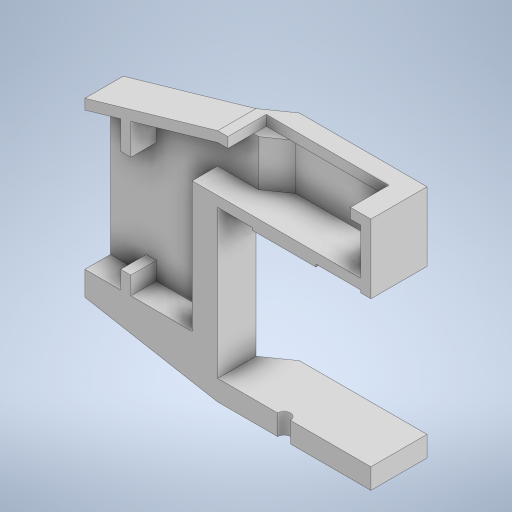
# Autodesk Inventor part: wirst 1 left
Saved by Autodesk Inventor 2023 (Build 270158000, 158)
## iProperties
Created: 2024-06-27
Part Number: wirst 1 left
Material: Generic
Document SubType Name: Modeling
Designer: Swoby
Density: 1 g/cm^3
Appearance: Default
Author: Swoby
Autodesk Inventor part; units mm, degrees
ref_plane "YZ Plane" through (0, 0, 0) normal (1, 0, 0) x (0, 1, 0)
ref_plane "XZ Plane" through (0, 0, 0) normal (0, 1, 0) x (-1, 0, 0)
ref_plane "XY Plane" through (0, 0, 0) normal (0, 0, 1) x (1, 0, 0)
sketch "Sketch1" plane through (0, 0, 0) normal (0, 0, 1) x (1, 0, 0)
  line L0 (-26, -31) -> (26, -31)
  line L1 (26, -31) -> (26, 31)
  line L2 (26, 31) -> (-26, 31)
  line L3 (-26, 31) -> (-26, -31)
  line L4 (-26, -31) -> (26, 31) construction
  line L5 (26, -31) -> (-26, 31) construction
  line L6 (-24, -23) -> (-24, -9) construction
  line L7 (-26, 31) -> (26, 46)
  line L8 (26, 46) -> (86, 46)
  line L9 (86, 46) -> (86, 19)
  line L10 (86, 19) -> (26, 19)
  point P0 (0, 0)
  dimension "d0" = 2
  dimension "d1" = 62
  dimension "d2" = 52
  dimension "d3" = 15
  dimension "d4" = 50
  dimension "d5" = 60
  constraints: 22 end point, 3 parallel, 3 perpendicular, 2 horizontal, 2 midpoint, 2 point on line
  measures "d0" distance between parallel lines of L3 L6
  measures "d1" distance of L2.end L0.start
  measures "d2" distance of L0.start L0.end
  measures "d3" distance of L1.end L7.end
  measures "d4" distance between parallel lines of L0 L10
  measures "d5" distance of L7.end L8.end
extrude "Extrusion1" add sketch "Sketch1" along normal blind 5
sketch "Sketch2" plane through (0, 0, 5) normal (0, 0, 1) x (1, 0, 0)
  line L0 (-29, 11.5) -> (-29, 6.5) construction
  line L1 (-29, 6.5) -> (-24, 6.5) construction
  line L2 (-24, 6.5) -> (-24, -20) construction
  line L3 (-24, -20) -> (-15, -20) construction
  line L4 (-15, -20) -> (-15, -27) construction
  line L5 (-15, -27) -> (-12, -27) construction
  line L6 (-12, -27) -> (-12, -20) construction
  line L7 (-12, -20) -> (16, -20) construction
  line L8 (16, -20) -> (16, 20) construction
  line L9 (16, 20) -> (11, 20) construction
  line L10 (11, 20) -> (11, 25) construction
  line L11 (11, 25) -> (8, 25) construction
  line L12 (8, 25) -> (8, 20) construction
  line L13 (8, 20) -> (-12, 20) construction
  line L14 (-12, 20) -> (-12, 27) construction
  line L15 (-12, 27) -> (-15, 27) construction
  line L16 (-15, 27) -> (-15, 20) construction
  line L17 (-15, 20) -> (-24, 20) construction
  line L18 (26, 46) -> (-26, 31) projected
  line L19 (-24, 20) -> (-24, 11.5) construction
  line L20 (-24, 11.5) -> (-29, 11.5) construction
  line L21 (-26, 31) -> (-26, -31) construction
  line L22 (-26, -31) -> (26, -31) construction
  line L23 (-12, 31.0385) -> (-12, 20)
  line L24 (-12, 20) -> (-8, 20)
  line L25 (-8, 20) -> (-8, 32.1923)
  line L26 (-26, 27) -> (26, 42)
  line L27 (-26, -27) -> (-12, -27)
  line L28 (-12, -27) -> (-12, -20)
  line L29 (-12, -20) -> (-8, -20)
  line L30 (-8, -20) -> (-8, -27)
  line L31 (-8, -27) -> (16, -27)
  line L32 (16, -27) -> (16, 20)
  line L33 (26, -31) -> (26, 19) projected
  line L34 (26, 24) -> (26, 19) construction
  line L35 (-26, 31) -> (-26, 27)
  line L36 (86, 46) -> (26, 46) projected
  line L37 (26, 46) -> (26, 42)
  line L38 (26, 42) -> (82, 42)
  line L39 (82, 42) -> (82, 19)
  line L40 (26, 19) -> (86, 19) projected
  line L41 (86, 19) -> (86, 46) projected
  line L42 (-26, -27) -> (-26, -31)
  line L43 (-26, -31) -> (26, -31)
  line L44 (16, 20) -> (16, 24)
  line L45 (16, 24) -> (26, 24)
  line L46 (26, 24) -> (82, 24)
  line L47 (26, 19) -> (26, 20)
  line L48 (26, 20) -> (82, 20)
  point P0 (0, 0)
  dimension "d8" = 3
  dimension "d9" = 3
  dimension "d10" = 3
  dimension "d11" = 7
  dimension "d12" = 54
  dimension "d13" = 7
  dimension "d14" = 5
  dimension "d15" = 5
  dimension "d16" = 2
  dimension "d17" = 9
  dimension "d18" = 8.5
  dimension "d19" = 4
  dimension "d20" = 5
  dimension "d21" = 5
  dimension "d22" = 40
  dimension "d23" = 4
  dimension "d25" = 4
  dimension "d26" = 10
  dimension "d27" = 4
  dimension "d28" = 4
  dimension "d36" = 1
  dimension "d37" = 4
  constraints: 84 end point, 16 point on line, 14 perpendicular, 12 parallel, 8 collinear, 2 horizontal, 2 vertical
  measures "d8" distance of L14.end L15.end
  measures "d9" distance of L10.end L11.end
  measures "d10" distance of L4.end L5.end
  measures "d11" distance of L15.end L16.end
  measures "d12" distance between parallel lines of L5 L15
  measures "d13" distance of L3.end L4.end
  measures "d14" distance between parallel lines of L13 L11
  measures "d15" distance of L8.end L9.end
  measures "d16" distance between parallel lines of L21 L2
  measures "d17" distance of L2.end L3.end
  measures "d18" distance of L17.end L19.end
  measures "d19" distance between parallel lines of L22 L5
  measures "d20" distance of L0.start L0.end
  measures "d21" distance of L19.end L0.start
  measures "d22" distance between parallel lines of L8 L2
  measures "d23" distance between parallel lines of L25 L23
  measures "d25" distance between parallel lines of L30 L6
  measures "d26" distance between parallel lines of L33 L32
  measures "d27" distance between parallel lines of L41 L39
  measures "d28" distance of L18.start L26.end
  measures "d36" distance of L33.end L47.end
  measures "d37" distance between parallel lines of L48 L46
extrude "Extrusion2" add sketch "Sketch2" along normal blind 10 contours L37 L26 L35 L18 | L36 L41 L40 L39 L38 L37 | L25 L24 L23 L26 | L39 L48 L47 L33 L43 L42 L27 L28 L29 L30 L31 L32 L44 L45 L46
sketch "Sketch3" plane through (0, 0, 15) normal (0, 0, 1) x (1, 0, 0)
  line L0 (-26, 27) -> (-12, 31.0385) projected
  line L1 (-12, 31.0385) -> (-12, 20) projected
  line L2 (-12, 20) -> (-8, 20) projected
  line L3 (-8, 20) -> (-8, 32.1923) projected
  line L4 (-8, 32.1923) -> (26, 42) projected
  line L5 (26, 42) -> (82, 42) projected
  line L6 (82, 42) -> (82, 24) projected
  line L7 (82, 19) -> (86, 19) projected
  line L8 (86, 19) -> (86, 46) projected
  line L9 (86, 46) -> (26, 46) projected
  line L10 (26, 46) -> (-26, 31) projected
  line L11 (-26, 31) -> (-26, 27) projected
  line L12 (30, 42) -> (78, 42)
  line L13 (78, 42) -> (78, 46)
  line L14 (78, 46) -> (30, 46)
  line L15 (30, 46) -> (30, 42)
  line L16 (82, 24) -> (16, 24) projected
  line L17 (16, 24) -> (16, -27) projected
  line L18 (16, -27) -> (-8, -27) projected
  line L19 (-8, -27) -> (-8, -20) projected
  line L20 (-8, -20) -> (-12, -20) projected
  line L21 (-12, -20) -> (-12, -27) projected
  line L22 (-12, -27) -> (-26, -27) projected
  line L23 (-26, -27) -> (-26, -31) projected
  line L24 (-26, -31) -> (26, -31) projected
  line L25 (26, -31) -> (26, 20) projected
  line L26 (26, 20) -> (82, 20) projected
  line L27 (82, 20) -> (82, 19) projected
  point P0 (0, 0)
  point P1 (30, 46)
  dimension "d31" = 4
  dimension "d32" = 4
  constraints: 8 end point, 2 parallel, 2 point on line, 1 horizontal, 1 perpendicular
  measures "d31" distance between parallel lines of L6 L13
  measures "d32" distance from line of L9.end L15
extrude "Extrusion3" cut sketch "Sketch3" against normal through all contours L9 L13 L5 L15
sketch "Sketch4" plane through (26, 20, 5) normal (0, -1, 0) x (1, 0, 0)
  line L0 (0, 10) -> (56, 10) projected
  arc A0 (13.5, 10) -> (38.5, 10) centre (26, 10) ccw
  line L1 (0, -5) -> (0, 10) projected
  line L2 (13.5, 10) -> (38.5, 10)
  point P0 (-26, -5)
  dimension "d38" = 25
  dimension "d39" = 26
  constraints: 3 point on line, 2 end point, 2 point on circle, 1 centre point
  measures "d38" diameter of A0
  measures "d39" distance from line of L1 A0.centre
sketch "Sketch5" plane through (26, 19, 0) normal (0, -1, 0) x (1, 0, 0)
  line L0 (0, 0) -> (60, 0) projected
  line L1 (60, 0) -> (60, -7)
  line L2 (60, -7) -> (10, -7)
  line L3 (10, -7) -> (0, 0)
  point P0 (-26, 0)
  dimension "d40" = 50
  dimension "d41" = 7
  constraints: 6 end point, 1 perpendicular, 1 vertical
  measures "d40" distance of L1.end L2.end
  measures "d41" distance of L0.end L1.end
extrude "Extrusion4" add sketch "Sketch5" against normal up to surface (27 mm away)
sketch "Sketch6" plane through (26, 19, 5) normal (0, -1, 0) x (1, 0, 0)
  line L0 (0, 0) -> (56, 0) projected
  line L1 (56, 0) -> (56, -8)
  line L2 (56, -8) -> (10, -8)
  line L3 (0, -5) -> (0, 10) projected
  line L4 (60, -12) -> (60, 10) projected
  line L5 (10, -12) -> (60, -12) projected
  line L6 (0, -5) -> (10, -12) projected
  line L7 (10, -8) -> (10, -12)
  line L8 (10, -8) -> (0, -1)
  point P0 (-26, -5)
  point P1 (35, -12)
  dimension "d44" = 4
  dimension "d45" = 4
  dimension "d47" = 4
  constraints: 8 end point, 2 vertical, 1 midpoint, 1 perpendicular, 1 point on line
  measures "d44" distance between parallel lines of L4 L1
  measures "d45" distance from line of point (35, -12) L2
  measures "d47" distance of L3.start L8.end
extrude "Extrusion5" cut sketch "Sketch6" against normal up to surface (1 mm away) contours L0 L1 L2 L8 L3
extrude "Extrusion6" add sketch "Sketch4" along normal up to surface (1 mm away)
sketch "Sketch8" plane through (30, 42, 5) normal (0, 1, 0) x (1, 0, 0)
  line L0 (0, 5) -> (48, 5) projected
  line L1 (0, 0) -> (0, 5) projected
  line L2 (48, 0) -> (0, 0) projected
  line L3 (48, 0) -> (48, 5) projected
  line L4 (-14, 0) -> (52, 0) projected
  line L5 (2, 0) -> (10.5714, 6)
  line L6 (10.5714, 6) -> (48, 6)
  line L7 (48, 6) -> (48, 0)
  line L8 (2, 0) -> (48, 0)
  line L9 (-4, 5) -> (6, 12) projected
  line L10 (48, 6) -> (52, 6)
  line L11 (52, 6) -> (52, 0)
  line L12 (52, 0) -> (48, 0)
  line L13 (48, 0) -> (48, 6)
  point P0 (-30, 5)
  point P1 (9.1429, 5)
  point P2 (2, 0)
  dimension "d57" = 2
  constraints: 16 end point, 3 parallel, 2 perpendicular, 1 collinear, 1 horizontal, 1 point on line
  measures "d57" distance from line of L1 L5.start
extrude "Extrusion8" cut sketch "Sketch8" against normal up to surface (18 mm away) contours L5 L6 L7 L0 | L0 L3 L2 L5 | L7 L10 L11 L4 L3
sketch "Sketch9" plane through (-26, -31, 0) normal (0, -1, 0) x (1, 0, 0)
  line L0 (62, -3) -> (52, 4) projected
  line L1 (52, 0) -> (52, 4) projected
  line L2 (52, 0) -> (62, -7) projected
  line L3 (62, -7) -> (112, -7) projected
  line L4 (112, -7) -> (112, 15) projected
  line L5 (108, 15) -> (112, 15) projected
  line L6 (108, 15) -> (108, -3) projected
  line L7 (108, -3) -> (62, -3) projected
  line L8 (52, 15) -> (65.5, 15) projected
  line L9 (65.5, 15) -> (90.5, 15) projected
  line L10 (90.5, 15) -> (108, 15) projected
  line L11 (0, 0) -> (52, 0) projected
  line L12 (52, 0) -> (52, 15) projected
  line L13 (0, 15) -> (52, 15) projected
  line L14 (0, 0) -> (0, 15) projected
  point P0 (26, 0)
extrude "Extrusion9" add sketch "Sketch9" along normal blind 15
sketch "Sketch10" plane through (0, 0, 15) normal (0, 0, 1) x (1, 0, 0)
  line L0 (26, -31) -> (86, -31)
  line L1 (86, -31) -> (86, -38)
  line L2 (86, -38) -> (26, -38)
  line L3 (26, -38) -> (26, -31)
  point P0 (0, 0)
  dimension "d62" = 7
  constraints: 8 end point, 2 parallel, 1 horizontal, 1 perpendicular
  measures "d62" distance between parallel lines of L2 L0
extrude "Extrusion10" cut sketch "Sketch10" against normal through all
sketch "Sketch11" plane through (0, 0, 15) normal (0, 0, 1) x (1, 0, 0)
  line L0 (-26, -46) -> (26, -46) projected
  line L1 (26, -46) -> (-26, -46)
  line L2 (-26, -46) -> (-26, -36.5)
  line L3 (26, -46) -> (-26, -36.5)
  point P0 (0, 0)
  dimension "d65" = 9.5
  constraints: 6 end point, 1 collinear, 1 perpendicular
  measures "d65" distance of L0.start L2.end
extrude "Extrusion11" cut sketch "Sketch11" against normal through all
sketch "Sketch12" plane through (26, -38, 15) normal (0, 1, 0) x (1, 0, 0)
  arc A0 (38.5, 0) -> (13.5, 0) centre (26, 0) ccw projected
  line L0 (13.5, 0) -> (38.5, 0) projected
  circle A1 centre (26, 0) radius 2.5
  point P0 (-26, 15)
  dimension "d68" = 5
  constraints: 1 centre point, 1 coincident
  measures "d68" diameter of A1
extrude "Extrusion12" cut sketch "Sketch12" against normal through all contours A1 L0 | L0 A1
equation "\"d45\" = d44"
body "Solid1"
